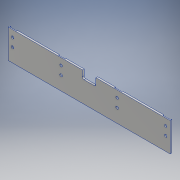
# Autodesk Inventor part: 앞뒷판_밑
Saved by Autodesk Inventor 2017 (Build 210142000, 142)
## iProperties
Part Number: 앞뒷판_밑
Material: 알루미늄 6061
Document SubType Name: Modeling
Designer: minom
Density: 2.7 g/cm^3
Appearance: 알루미늄 - 평지
Mass: 44.0581 g
Surface Area: 195.771 cm^2
Volume: 16.3178 cm^3
Author: minom
Autodesk Inventor part; units mm, degrees
ref_plane "YZ Plane" through (0, 0, 0) normal (1, 0, 0) x (0, 1, 0)
ref_plane "XZ Plane" through (0, 0, 0) normal (0, 1, 0) x (-1, 0, 0)
ref_plane "XY Plane" through (0, 0, 0) normal (0, 0, 1) x (1, 0, 0)
sketch "스케치1" plane through (0, 0, 0) normal (0, 1, 0) x (-1, 0, 0)
  line L0 (0, 0) -> (-270, 0)
  line L1 (-270, 0) -> (-270, -34)
  line L2 (-270, -34) -> (0, -34)
  line L3 (0, -34) -> (0, 0)
  dimension "d0" = 270
  dimension "d1" = 34
  constraints: 8 end point, 2 parallel, 1 horizontal, 1 perpendicular
  measures "d0" distance of L2.end L1.end
  measures "d1" distance of L1.end L0.end
extrude "돌출1" add sketch "스케치1" along normal blind 2
sketch "스케치2" plane through (0, 2, 0) normal (0, 1, 0) x (1, 0, 0)
  line L0 (0, 0) -> (270, 0) projected
  line L1 (0, 34) -> (0, 0) projected
  line L2 (270, 34) -> (0, 34) projected
  line L3 (270, 0) -> (270, 34) projected
  line L4 (270, 0) -> (270, 34) projected
  line L5 (41, 34) -> (41, 0)
  line L6 (41, 34) -> (49.2, 34)
  line L7 (49.2, 34) -> (49.2, 0)
  line L8 (0, 0) -> (270, 0) projected
  line L9 (230, 34) -> (229, 34)
  line L10 (229, 34) -> (220.8, 34)
  line L11 (220.8, 34) -> (220.8, 0)
  line L12 (229, 34) -> (229, 0)
  line L13 (1, 34) -> (1, 0)
  line L14 (9.2, 34) -> (9.2, 0)
  line L15 (269, 34) -> (269, 0)
  line L16 (260.8, 34) -> (260.8, 0)
  line L17 (1, 0) -> (9.2, 0)
  line L18 (260.8, 0) -> (269, 0)
  line L19 (229, 0) -> (220.8, 0)
  line L20 (41, 0) -> (49.2, 0)
  line L21 (1, 34) -> (9.2, 34)
  line L22 (270, 34) -> (0, 34) projected
  line L23 (260.8, 34) -> (269, 34)
  point P0 (285, 0)
  dimension "d4" = 40
  dimension "d7" = 8.2
  dimension "d8" = 1
  dimension "d9" = 8.2
  dimension "d17" = 1
  dimension "d18" = 8.2
  dimension "d19" = 1
  dimension "d20" = 8.2
  constraints: 34 end point, 5 collinear, 5 perpendicular, 2 point on line, 2 vertical, 1 horizontal, 8 other
  measures "d4" distance of L2.start L9.start
  measures "d7" distance of L5.start L6.end
  measures "d8" distance of L9.start L9.end
  measures "d9" distance of L9.end L10.end
  measures "d17" distance between parallel lines of L3 L15
  measures "d18" distance between parallel lines of L15 L16
  measures "d19" distance between parallel lines of L13 L1
  measures "d20" distance between parallel lines of L14 L13
extrude "돌출4" cut sketch "스케치2" against normal blind 1 contours L13 L2 L14 L0 | L5 L2 L7 L0 | L11 L2 L12 L0 | L16 L2 L15 L0
sketch "스케치4" plane through (0, 0, 0) normal (0, -1, 0) x (1, 0, 0)
  line L0 (0, 0) -> (270, 0) projected
  line L1 (0, -34) -> (0, 0) projected
  line L2 (270, -34) -> (0, -34) projected
  line L3 (270, 0) -> (270, -34) projected
  line L4 (127, 0) -> (143, 0)
  line L5 (143, 0) -> (143, -7)
  line L6 (141, -9) -> (129, -9)
  line L7 (127, -7) -> (127, 0)
  line L8 (0, -34) -> (0, 0) projected
  line L9 (270, 0) -> (270, -34) projected
  arc A0 (127, -7) -> (129, -9) centre (129, -7) ccw
  arc A1 (141, -9) -> (143, -7) centre (141, -7) ccw
  point P0 (143, -9)
  point P1 (127, -9)
  dimension "d23" = 9
  dimension "d24" = 127
  dimension "d25" = 127
  dimension "d54" = 2
  constraints: 8 end point, 5 point on line, 4 point on circle, 4 tangent, 2 centre point, 2 parallel, 1 equal radius, 1 horizontal, 1 perpendicular
  measures "d23" distance of L4.end point (143, -9)
  measures "d24" distance between parallel lines of L7 L8
  measures "d25" distance between parallel lines of L9 L5
  measures "d54" radius of A0
extrude "돌출5" cut sketch "스케치4" against normal blind 10 contours L0 L5 A1 L6 A0 L7
sketch "스케치5" plane through (0, 0, 0) normal (0, -1, 0) x (1, 0, 0)
  line L0 (9.2, 0) -> (1, 0) projected
  line L1 (9.2, -34) -> (9.2, 0) projected
  line L2 (1, -34) -> (9.2, -34) projected
  line L3 (1, 0) -> (1, -34) projected
  line L4 (49.2, 0) -> (41, 0) projected
  line L5 (49.2, -34) -> (49.2, 0) projected
  line L6 (41, -34) -> (49.2, -34) projected
  line L7 (41, 0) -> (41, -34) projected
  line L8 (229, 0) -> (220.8, 0) projected
  line L9 (229, -34) -> (229, 0) projected
  line L10 (220.8, -34) -> (229, -34) projected
  line L11 (220.8, 0) -> (220.8, -34) projected
  line L12 (269, 0) -> (260.8, 0) projected
  line L13 (269, -34) -> (269, 0) projected
  line L14 (260.8, -34) -> (269, -34) projected
  line L15 (260.8, 0) -> (260.8, -34) projected
  circle A0 centre (5.1, -8) radius 1.5
  circle A1 centre (5.1, -18) radius 1.5
  circle A2 centre (45.1, -8) radius 1.5
  circle A3 centre (45.1, -18) radius 1.5
  circle A4 centre (224.9, -18) radius 1.5
  circle A5 centre (224.9, -8) radius 1.5
  circle A6 centre (264.9, -8) radius 1.5
  circle A7 centre (264.9, -18) radius 1.5
  point P0 (0, 0)
  dimension "d28" = 3
  dimension "d29" = 3
  dimension "d30" = 3
  dimension "d31" = 4.1
  dimension "d32" = 4.1
  dimension "d33" = 4.1
  dimension "d34" = 4.1
  dimension "d35" = 4.1
  dimension "d36" = 4.1
  dimension "d37" = 4.1
  dimension "d38" = 4.1
  dimension "d39" = 8
  dimension "d40" = 16
  dimension "d41" = 16
  dimension "d42" = 8
  dimension "d43" = 8
  dimension "d44" = 3
  dimension "d45" = 16
  dimension "d46" = 3
  dimension "d47" = 16
  dimension "d48" = 8
  dimension "d49" = 3
  dimension "d50" = 3
  dimension "d51" = 3
  constraints: 8 centre point
  measures "d28" diameter of A0
  measures "d29" diameter of A1
  measures "d30" diameter of A6
  measures "d31" distance from line of L3 A0.centre
  measures "d32" distance from line of L1 A1.centre
  measures "d33" distance from line of L5 A3.centre
  measures "d34" distance from line of L7 A2.centre
  measures "d35" distance from line of L11 A5.centre
  measures "d36" distance from line of L9 A4.centre
  measures "d37" distance from line of L15 A7.centre
  measures "d38" distance from line of L13 A6.centre
  measures "d39" distance from line of L0 A0.centre
  measures "d40" distance from line of L2 A1.centre
  measures "d41" distance from line of L6 A3.centre
  measures "d42" distance from line of L4 A2.centre
  measures "d43" distance from line of L8 A5.centre
  measures "d44" diameter of A5
  measures "d45" distance from line of L10 A4.centre
  measures "d46" diameter of A4
  measures "d47" distance from line of L14 A7.centre
  measures "d48" distance from line of L12 A6.centre
  measures "d49" diameter of A7
  measures "d50" diameter of A2
  measures "d51" diameter of A3
extrude "돌출6" cut sketch "스케치5" against normal blind 10 contours A0 | A1 | A2 | A3 | A4 | A5 | A6 | A7
sketch "스케치6" plane through (0, 2, 0) normal (0, 1, 0) x (1, 0, 0)
  line L0 (143, 7) -> (143, 0) projected
  line L1 (143, 0) -> (220.8, 0) projected
  line L2 (220.8, 0) -> (220.8, 34) projected
  line L3 (220.8, 34) -> (49.2, 34) projected
  line L4 (49.2, 34) -> (49.2, 0) projected
  line L5 (127, 0) -> (127, 7) projected
  arc A0 (129, 9) -> (127, 7) centre (129, 7) ccw projected
  line L6 (129, 9) -> (141, 9) projected
  arc A1 (143, 7) -> (141, 9) centre (141, 7) ccw projected
  circle A2 centre (264.9, 8) radius 1.5 projected
  circle A3 centre (224.9, 18) radius 1.5 projected
  circle A4 centre (45.1, 8) radius 1.5 projected
  circle A5 centre (5.1, 8) radius 1.5 projected
  circle A6 centre (5.1, 18) radius 1.5 projected
  circle A7 centre (45.1, 18) radius 1.5 projected
  circle A8 centre (224.9, 8) radius 1.5 projected
  circle A9 centre (264.9, 18) radius 1.5 projected
  line L7 (143, 0) -> (143, 7) projected
  arc A10 (141, 9) -> (143, 7) centre (141, 7) ccw projected
  line L8 (141, 9) -> (129, 9) projected
  arc A11 (127, 7) -> (129, 9) centre (129, 7) ccw projected
  line L9 (127, 7) -> (127, 0) projected
  line L10 (0, 0) -> (127, 0) projected
  line L11 (0, 34) -> (0, 0) projected
  line L12 (270, 34) -> (0, 34) projected
  line L13 (270, 0) -> (270, 34) projected
  line L14 (49.2, 0) -> (127, 0) projected
  line L15 (98, 34) -> (106.2, 34)
  line L16 (106.2, 34) -> (106.2, 0)
  line L17 (106.2, 0) -> (98, 0)
  line L18 (98, 0) -> (98, 34)
  line L19 (220.8, 34) -> (49.2, 34) projected
  line L20 (143, 0) -> (220.8, 0) projected
  line L21 (163.8, 34) -> (172, 34)
  line L22 (172, 34) -> (172, 0)
  line L23 (172, 0) -> (163.8, 0)
  line L24 (163.8, 0) -> (163.8, 34)
  line L25 (229, 34) -> (229, 0) projected
  line L26 (229, 0) -> (260.8, 0) projected
  line L27 (260.8, 0) -> (260.8, 34) projected
  line L28 (260.8, 34) -> (229, 34) projected
  line L29 (41, 0) -> (41, 34) projected
  line L30 (41, 34) -> (9.2, 34) projected
  line L31 (9.2, 34) -> (9.2, 0) projected
  line L32 (9.2, 0) -> (41, 0) projected
  line L33 (1, 0) -> (1, 34) projected
  line L34 (1, 34) -> (0, 34) projected
  line L35 (0, 34) -> (0, 0) projected
  line L36 (0, 0) -> (1, 0) projected
  line L37 (269, 34) -> (269, 0) projected
  line L38 (269, 0) -> (270, 0) projected
  line L39 (270, 0) -> (270, 34) projected
  line L40 (270, 34) -> (269, 34) projected
  line L41 (49.2, 0) -> (127, 0) projected
  line L42 (143, 0) -> (270, 0) projected
  point P0 (163, 0)
  dimension "d55" = 8.2
  dimension "d56" = 8.2
  dimension "d57" = 98
  dimension "d58" = 98
  constraints: 16 end point, 4 parallel, 4 point on line, 2 horizontal, 2 perpendicular
  measures "d55" distance of L16.end L17.end
  measures "d56" distance of L22.end L23.end
  measures "d57" distance between parallel lines of L18 L11
  measures "d58" distance between parallel lines of L22 L13
extrude "돌출7" cut sketch "스케치6" against normal blind 1 contours L24 L3 L22 L1 | L16 L10 L18 L3
sketch "스케치7" plane through (0, 1, 0) normal (0, 1, 0) x (1, 0, 0)
  line L0 (106.2, 34) -> (106.2, 0) projected
  line L1 (98, 34) -> (106.2, 34) projected
  line L2 (98, 0) -> (98, 34) projected
  line L3 (106.2, 0) -> (98, 0) projected
  line L4 (172, 34) -> (172, 0) projected
  line L5 (163.8, 34) -> (172, 34) projected
  line L6 (163.8, 0) -> (163.8, 34) projected
  line L7 (172, 0) -> (163.8, 0) projected
  circle A0 centre (102.1, 8) radius 1.5
  circle A1 centre (102.1, 18) radius 1.5
  circle A2 centre (167.9, 18) radius 1.5
  circle A3 centre (167.9, 8) radius 1.5
  point P0 (0, 0)
  dimension "d61" = 3
  dimension "d62" = 3
  dimension "d63" = 3
  dimension "d64" = 3
  dimension "d65" = 4.1
  dimension "d66" = 4.1
  dimension "d67" = 4.1
  dimension "d68" = 4.1
  dimension "d69" = 8
  dimension "d71" = 8
  dimension "d75" = 16
  dimension "d76" = 16
  constraints: 4 centre point
  measures "d61" diameter of A0
  measures "d62" diameter of A1
  measures "d63" diameter of A2
  measures "d64" diameter of A3
  measures "d65" distance from line of A1.centre L2
  measures "d66" distance from line of L0 A0.centre
  measures "d67" distance from line of A3.centre L6
  measures "d68" distance from line of L4 A2.centre
  measures "d69" distance from line of L3 A0.centre
  measures "d71" distance from line of L7 A3.centre
  measures "d75" distance from line of L1 A1.centre
  measures "d76" distance from line of L5 A2.centre
extrude "돌출8" cut sketch "스케치7" against normal blind 1 contours A0 | A1 | A2 | A3
sketch "스케치8" plane through (0, 2, 0) normal (0, 1, 0) x (1, 0, 0)
  line L0 (230, 0) -> (230, 33)
  line L1 (40, 0) -> (40, 33)
  line L2 (230, 0) -> (270, 0)
  line L3 (270, 0) -> (270, 34)
  line L4 (270, 34) -> (230, 34)
  line L5 (230, 34) -> (230, 0)
  line L6 (1, 34) -> (0, 34) projected
  line L7 (40, 0) -> (0, 0)
  line L8 (0, 0) -> (0, 34)
  line L9 (0, 34) -> (40, 34)
  line L10 (40, 34) -> (40, 0)
  constraints: 20 end point, 4 parallel, 2 horizontal, 2 perpendicular
extrude "돌출9" cut sketch "스케치8" against normal blind 10
